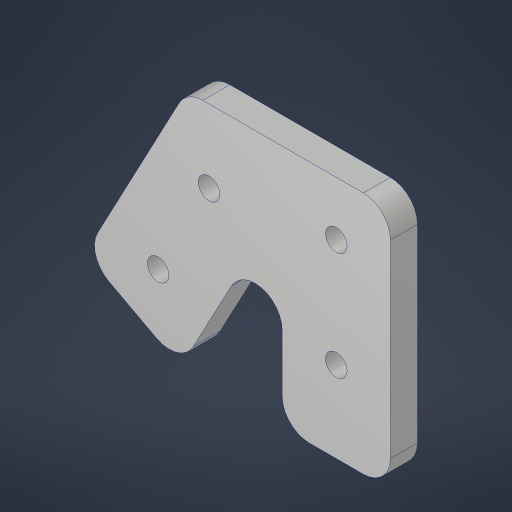
# Autodesk Inventor part: CL4-009
Saved by Autodesk Inventor 2023.4 (Build 274418000, 418)
## iProperties
Created: 2025-02-04
Part Number: CL4-009
Material: Aluminum 6061
Document SubType Name: Modeling
Designer: brand
Density: 2.7 g/cm^3
Appearance: Aluminum - Flat
Author: brand
Autodesk Inventor part; units mm, degrees
ref_plane "YZ Plane" through (0, 0, 0) normal (1, 0, 0) x (0, 1, 0)
ref_plane "XZ Plane" through (0, 0, 0) normal (0, 1, 0) x (-1, 0, 0)
ref_plane "XY Plane" through (0, 0, 0) normal (0, 0, 1) x (1, 0, 0)
sketch "Sketch1" plane through (0, 0, 0) normal (0, 0, 1) x (1, 0, 0)
  line L0 (-12.7, 0) -> (12.7, 0) construction
  line L1 (12.7, 0) -> (12.7, -57.15)
  line L2 (12.7, -57.15) -> (-12.7, -57.15)
  line L3 (-12.7, -57.15) -> (-12.7, 0) construction
  line L4 (-35.1269, 0) -> (-12.7, -11.9246) construction
  line L5 (-12.7, -11.9246) -> (-36.5492, -56.7783)
  line L6 (-36.5492, -56.7783) -> (-58.976, -44.8537)
  line L7 (-58.976, -44.8537) -> (-35.1269, 0)
  line L8 (-23.9134, -5.9623) -> (-47.7626, -50.816) construction
  line L9 (-35.1269, 0) -> (12.7, 0)
  line L10 (-12.7, -11.9246) -> (-12.7, -57.15)
  point P0 (0, 0)
  point P1 (0, 0)
  point P2 (-29.8757, -17.1757)
  point P3 (-41.8003, -39.6026)
  point P4 (0, -12.7)
  point P5 (0, -38.1)
  dimension "d0" = 25.4
  dimension "d1" = 25.4
  dimension "d2" = 28
  dimension "d3" = 50.8
  dimension "d4" = 25.4
  dimension "d5" = 12.7
  dimension "d6" = 25.4
  dimension "d7" = 12.7
  dimension "d8" = 57.15
  constraints: 22 end point, 4 perpendicular, 3 midpoint, 3 parallel, 3 point on line, 2 horizontal, 2 vertical alignment, 1 coincident, 1 horizontal alignment, 1 vertical
  measures "d0" distance of L1.end L2.end
  measures "d1" distance of L4.start L4.end
  measures "d2" angle of L3 L5
  measures "d3" distance of L8.start L8.end
  measures "d4" distance of point (-41.8, -39.603) point (-29.876, -17.176)
  measures "d5" distance from line of L4 point (-29.876, -17.176)
  measures "d6" distance of point (0, -38.1) point (0, -12.7)
  measures "d7" distance of point (0, 0) point (0, -12.7)
  measures "d8" distance of L0.end L1.end
extrude "Extrusion1" add sketch "Sketch1" against normal blind 6.35
hole "Hole1" at (-29.8757, -17.1757, 0) at (-41.8003, -39.6026, 0) at (0, -12.7, 0) at (0, -38.1, 0) direction (0, 0, -1) diameter 5.1054 end through all clearance for "Flat Head Machine Screw (82)" size "#10" standard "Ansi Unified Screw Threads"
fillet "Fillet1" radius 6.35 7 edges at (12.7, 0, -3.175) (12.7, -57.15, -3.175) (-12.7, -57.15, -3.175) (-12.7, -11.9246, -3.175) (-36.5492, -56.7783, -3.175) (-58.976, -44.8537, -3.175) (-35.1269, 0, -3.175)
body "Solid1"
